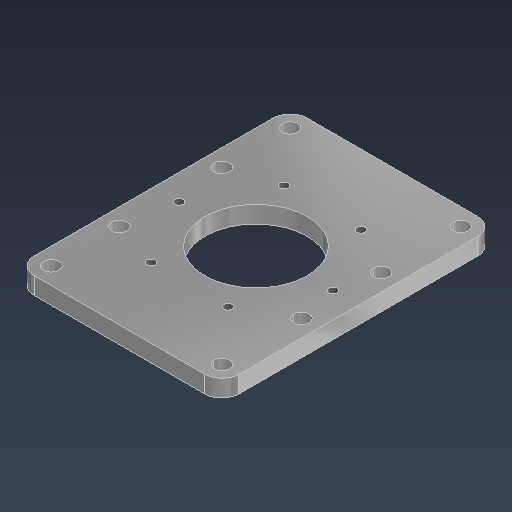
# Autodesk Inventor part: P017-Carter_chapeau
Saved by Autodesk Inventor 2021.3 (Build 253353000, 353)
## iProperties
Created: 2022-04-01
Part Number: P017-Carter_chapeau
Material: Aluminium
Document SubType Name: Modeling
Designer: remi
Density: 2.7 g/cm^3
Appearance: Aluminum - Dark
Mass: 69.432 g
Surface Area: 131.539 cm^2
Volume: 25.7156 cm^3
Author: remi
Autodesk Inventor part; units mm, degrees
ref_plane "YZ Plane" through (0, 0, 0) normal (1, 0, 0) x (0, 1, 0)
ref_plane "XZ Plane" through (0, 0, 0) normal (0, 1, 0) x (-1, 0, 0)
ref_plane "XY Plane" through (0, 0, 0) normal (0, 0, 1) x (1, 0, 0)
sketch "Sketch2" plane through (0, 0, 0) normal (0, 0, 1) x (1, 0, 0)
  arc A0 (30, 25) -> (25, 30) centre (25, 25) ccw projected
  line L0 (25, 30) -> (-25, 30) projected
  arc A1 (-25, 30) -> (-30, 25) centre (-25, 25) ccw projected
  line L1 (-30, 25) -> (-30, -45) projected
  arc A2 (-30, -45) -> (-25, -50) centre (-25, -45) ccw projected
  line L2 (-25, -50) -> (25, -50) projected
  arc A3 (25, -50) -> (30, -45) centre (25, -45) ccw projected
  line L3 (30, -45) -> (30, 25) projected
  circle A4 centre (25, 1.6667) radius 1.621 construction
  circle A5 centre (-25, -25) radius 1.621 construction
  circle A6 centre (25, 25) radius 1.621 construction
  circle A7 centre (-25, -45) radius 1.621 construction
  circle A8 centre (25, -45) radius 1.621 construction
  circle A9 centre (-25, 25) radius 1.621 construction
  circle A10 centre (-25, 5) radius 1.621 construction
  circle A11 centre (25, -21.6667) radius 1.621 construction
  line L4 (20, -40) -> (-20, -40) construction
  line L5 (-20, -40) -> (-20, 20) construction
  line L6 (-20, 20) -> (20, 20) construction
  line L7 (20, 20) -> (20, -40) construction
  point P0 (0, 0)
extrude "Extrusion1" add sketch "Sketch2" along normal blind 5
sketch "Sketch3" plane through (0, 0, 5) normal (0, 0, 1) x (1, 0, 0)
  circle A0 centre (0, -10) radius 15
  line L0 (25, 30) -> (-25, 30) construction
  arc A1 (-25, 30) -> (-30, 25) centre (-25, 25) ccw construction
  line L1 (-30, 25) -> (-30, -45) construction
  arc A2 (-30, -45) -> (-25, -50) centre (-25, -45) ccw construction
  line L2 (-25, -50) -> (25, -50) construction
  arc A3 (25, -50) -> (30, -45) centre (25, -45) ccw construction
  line L3 (30, -45) -> (30, 25) construction
  arc A4 (30, 25) -> (25, 30) centre (25, 25) ccw construction
  line L4 (-25, -45) -> (25, 25) construction
  line L5 (25, -45) -> (-25, 25) construction
  dimension "d6" = 30
  constraints: 4 end point, 2 midpoint, 1 centre point, 1 coincident
  measures "d6" diameter of A0
extrude "Extrusion2" cut sketch "Sketch3" against normal blind 5
sketch "Sketch6" plane through (0, 0, 5) normal (0, 0, 1) x (1, 0, 0)
  line L0 (30, -45) -> (30, 25) construction
  line L1 (25, 30) -> (-25, 30) construction
  line L2 (-30, 25) -> (-30, -45) construction
  line L3 (-25, -50) -> (25, -50) construction
  line L4 (20, -40) -> (-20, -40) construction
  line L5 (-20, -40) -> (-20, 20) construction
  line L6 (-20, 20) -> (20, 20) construction
  line L7 (20, 20) -> (20, -40) construction
  circle A0 centre (25, -21.6667) radius 1.621 construction
  circle A1 centre (-25, 5) radius 1.621 construction
  circle A2 centre (-25, 25) radius 1.621 construction
  circle A3 centre (25, -45) radius 1.621 construction
  circle A4 centre (-25, -45) radius 1.621 construction
  circle A5 centre (25, 25) radius 1.621 construction
  circle A6 centre (-25, -25) radius 1.621 construction
  circle A7 centre (25, 1.6667) radius 1.621 construction
  arc A8 (-30, -45) -> (-25, -50) centre (-25, -45) ccw projected
  arc A9 (25, -50) -> (30, -45) centre (25, -45) ccw projected
  arc A10 (30, 25) -> (25, 30) centre (25, 25) ccw projected
  arc A11 (-25, 30) -> (-30, 25) centre (-25, 25) ccw projected
hole "Hole3" at (-25, -45, 5) at (-25, -25, 5) at (-25, 5, 5) at (-25, 25, 5) at (25, 25, 5) at (25, 1.6667, 5) at (25, -21.6667, 5) at (25, -45, 5) direction (0, 0, -1) diameter 4.5 end through all clearance for "Flat Head Machine Screw" size "M4" standard "Ansi Metric M Profile"
sketch "Sketch7" plane through (0, 0, 5) normal (0, 0, 1) x (1, 0, 0)
  circle A0 centre (0, -10) radius 25 construction
  circle A1 centre (0, -10) radius 20 construction
  circle A2 centre (0, -10) radius 22.5 construction
  circle A3 centre (0, -10) radius 15 construction
  line L0 (-58.8, 0) -> (58.8, 0) construction
  line L1 (42, -10) -> (-42, -10) construction
  point P0 (-22.5, -10)
  point P1 (-11.25, -29.4856)
  point P2 (11.25, -29.4856)
  point P3 (22.5, -10)
  point P4 (11.25, 9.4856)
  point P5 (-11.25, 9.4856)
  dimension "d43" = 45
  dimension "d41" = 50
  dimension "d42" = 40
  dimension "d46" = 360
  constraints: 3 coincident, 2 end point, 1 horizontal, 1 horizontal alignment, 1 midpoint, 1 point on line, 10 other
  measures "d41" diameter of A0
  measures "d42" diameter of A1
hole "Hole4" at (-22.5, -10, 5) at (-11.25, -29.4856, 5) at (11.25, -29.4856, 5) at (22.5, -10, 5) at (11.25, 9.4856, 5) at (-11.25, 9.4856, 5) direction (0, 0, -1) diameter 2.459 depth 4 thread size "M3x0.5" class "6H" standard "ISO Metric profile"
equation "\"d43\" = 0.5 * d41 + 0.5 * d42"
body "Solid1"
